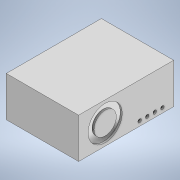
# Autodesk Inventor part: pms5003
Saved by Autodesk Inventor 2022 (Build 260153000, 153)
## iProperties
Created: 2023-04-22
Part Number: pms5003
Material: Generic
Document SubType Name: Modeling
Designer: User
Density: 1 g/cm^3
Appearance: Default
Author: User
Autodesk Inventor part; units mm, degrees
ref_plane "YZ Plane" through (0, 0, 0) normal (1, 0, 0) x (0, 1, 0)
ref_plane "XZ Plane" through (0, 0, 0) normal (0, 1, 0) x (-1, 0, 0)
ref_plane "XY Plane" through (0, 0, 0) normal (0, 0, 1) x (1, 0, 0)
sketch "Sketch1" plane through (0, 0, 0) normal (0, 1, 0) x (-1, 0, 0)
  line L0 (0, 0) -> (-38.17, 0)
  line L1 (-38.17, 0) -> (-38.17, -50.2)
  line L2 (-38.17, -50.2) -> (0, -50.2)
  line L3 (0, -50.2) -> (0, 0)
  dimension "d0" = 38.17
  dimension "d1" = 50.2
  constraints: 8 end point, 2 parallel, 1 coincident, 1 horizontal, 1 perpendicular
  measures "d0" distance of L2.end L1.end
  measures "d1" distance of L1.end L0.end
extrude "Extrusion1" add sketch "Sketch1" along normal blind 21.18
shell "Shell1" thickness 1 removed faces 0
sketch "Sketch2" plane through (38.17, 0, 0) normal (1, 0, 0) x (0, 0, -1)
  circle A0 centre (14, 10.59) radius 9
  line L0 (0, 0) -> (0, 21.18) projected
  circle A1 centre (14, 10.59) radius 5.9
  circle A2 centre (32.2, 2.5) radius 0.9353
  circle A3 centre (36.2, 2.5) radius 0.9353
  circle A4 centre (40.2, 2.5) radius 0.9353
  circle A5 centre (44.2, 2.5) radius 0.9353
  line L1 (50.2, 0) -> (50.2, 21.18) projected
  line L2 (0, 0) -> (50.2, 0) projected
  point P0 (0, 10.59)
  dimension "d4" = 18
  dimension "d5" = 14
  dimension "d6" = 11.8
  dimension "d9" = 6
  dimension "d10" = 2.5
  dimension "d11" = 4
  dimension "d12" = 4
  dimension "d13" = 4
  constraints: 6 centre point, 4 horizontal alignment, 3 equal radius, 1 coincident, 1 midpoint
  measures "d4" diameter of A0
  measures "d5" distance from line of L0 A0.centre
  measures "d6" diameter of A1
  measures "d9" distance from line of L1 A5.centre
  measures "d10" distance from line of L2 A5.centre
  measures "d11" distance of A4.centre A5.centre
  measures "d12" distance of A3.centre A4.centre
  measures "d13" distance of A2.centre A3.centre
extrude "Extrusion2" cut sketch "Sketch2" against normal blind 4
sketch "Sketch3" plane through (0, 0, -50.2) normal (-1, 0, 0) x (0, 0, 1)
  line L0 (27.9, 12.6) -> (44.9, 12.6)
  line L1 (44.9, 12.6) -> (44.9, 7.6)
  line L2 (44.9, 7.6) -> (27.9, 7.6)
  line L3 (27.9, 7.6) -> (27.9, 12.6)
  line L4 (0, 0) -> (50.2, 0) projected
  dimension "d15" = 5
  dimension "d16" = 17
  dimension "d17" = 7.6
  dimension "d18" = 5.3
  constraints: 8 end point, 2 parallel, 1 horizontal, 1 perpendicular
  measures "d15" distance between parallel lines of L2 L0
  measures "d16" distance of L1.end L2.end
  measures "d17" distance between parallel lines of L4 L2
  measures "d18" horizontal distance of L4.end L1.end
extrude "Extrusion3" cut sketch "Sketch3" against normal blind 4
equation "\"d7\" = d13"
equation "\"d19\" = d13"
body "Solid1"
